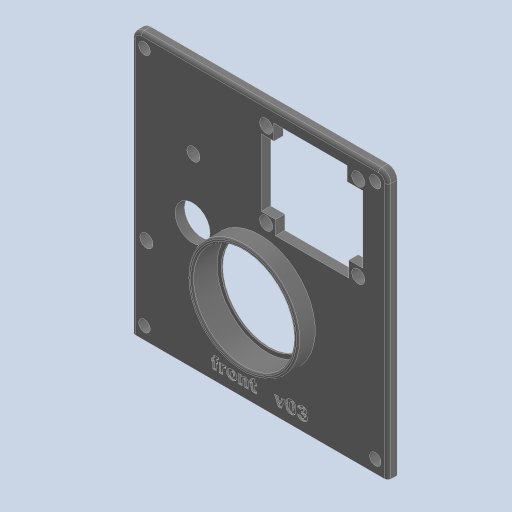
# Autodesk Inventor part: door_front_03b
Saved by Autodesk Inventor 2024.4 (Build 284460030, 460C)
## iProperties
Created: 2026-07-13
Part Number: door_front_03b
Material: Generic
Document SubType Name: Modeling
Designer: tooles01
Density: 1 g/cm^3
Appearance: Gray
d0: 3.000 mm
d1: 0.00 deg
d3: 32.500 mm
d4: 35.500 mm
d6: 0.00 deg
d11: 29.750 mm
d13: 0.00 deg
d14: 3.700 mm
d0_1: 36.000 mm
d3_1: 4.900 mm
d4_1: 3.000 mm
d5_1: 10.000 mm
d6_1: 2.000 mm
d7: 2.000 mm
d21: 30.000 mm
d22: 82.000 mm
d23: 4.000 mm
d24: 4.000 mm
d25: 4.000 mm
d26: 4.200 mm
d27: 35.000 mm
d28: 3.000 mm
d29: 4.900 mm
d32: 6.500 mm
d33: 2.000 mm
d34: 2.000 mm
d35: 10.000 mm
d37: 36.000 mm
d38: 2.000 mm
d39: 4.900 mm
d41: 4.200 mm
d48: 1.000 ul
d52: 0.00 deg
d53: 3.000 mm
d54: 34.500 mm
d55: 32.000 mm
d56: 3.000 mm
d57: 2.500 mm
d58: 27.000 mm
d59: 19.000 mm
d60: 7.000 mm
d61: 4.200 mm
d68: 55.000 mm
d69: 3.000 mm
d70: 1.000 mm
d71: 0.500 mm
d72: 40.000 mm
d73: 0.500 mm
d75: 5.000 mm
door_diameter: 36.000 mm
axle_width: 4.900 mm
axle_height: 3.100 mm
handle_height: 10.000 mm
spacing_height: 2.000 mm
spacing_width: 2.000 mm
door_diameter_1: 36.000 mm
handle_height_1: 10.000 mm
spacing_width_1: 2.000 mm
door_spacing_width_1: 2.000 mm
door_handle_height_1: 10.000 mm
door_door_diameter_1: 36.000 mm
door_axle_width_1: 4.900 mm
door_spacing_height_1: 2.000 mm
door_axle_width_2: 4.900 mm
door_axle_height_1: 3.100 mm
door_spacing_height_2: 2.000 mm
d76: 4.000 mm
d77: 9.200 mm
d78: 1.000 mm
d81: 1.000 mm
d85: 29.500 mm
d88: 27.000 mm
M3_heatset: 4.200 mm
tube_cover_length: 8.500 mm
tube_stopper_thickness: 0.500 mm
Author: tooles01
Autodesk Inventor part; units mm, degrees
ref_plane "YZ Plane" through (0, 0, 0) normal (1, 0, 0) x (0, 1, 0)
ref_plane "XZ Plane" through (0, 0, 0) normal (0, 1, 0) x (-1, 0, 0)
ref_plane "XY Plane" through (0, 0, 0) normal (0, 0, 1) x (1, 0, 0)
derived "door_03.ipt"
sketch "Sketch1: base" plane through (0, 0, 0) normal (0, 0, 1) x (1, 0, 0)
  line L0 (-41, 85) -> (41, 85)
  line L1 (41, 85) -> (41, 0)
  line L2 (41, 0) -> (-41, 0)
  line L3 (-41, 0) -> (-41, 85)
  circle A0 centre (0, 30) radius 16.25
  line L4 (-37, 81) -> (37, 81) construction
  line L5 (37, 81) -> (37, 4) construction
  line L6 (37, 4) -> (-37, 4) construction
  line L7 (-37, 4) -> (-37, 81) construction
  point P0 (0, 0)
  point P1 (0, 0)
  point P2 (0, 4)
  dimension "d3" = 32.5
  dimension "d21" = 30
  dimension "d22" = 82
  dimension "d23" = 4
  dimension "d24" = 4
  dimension "d25" = 4
  dimension "d68" = 55
  constraints: 16 end point, 6 perpendicular, 5 coincident, 2 horizontal, 2 midpoint, 2 vertical alignment, 1 centre point
  measures "d3" diameter of A0
  measures "d21" distance from line of L2 A0.centre
  measures "d22" distance of L1.end L2.end
  measures "d23" distance between parallel lines of L2 L6
  measures "d24" distance between parallel lines of L3 L7
  measures "d25" distance between parallel lines of L0 L4
  measures "d68" distance from line of L0 A0.centre
sketch "Sketch2: tube cover/stopper" plane through (0, 0, 0) normal (0, 0, 1) x (1, 0, 0)
  circle A0 centre (0, 30) radius 17.75
  circle A1 centre (0, 30) radius 14.875
  circle A2 centre (0, 30) radius 16.25 projected
  point P0 (0, 0)
  dimension "d4" = 35.5
  dimension "d11" = 29.75
  constraints: 3 coincident, 2 centre point
  measures "d4" diameter of A0
  measures "d11" diameter of A1
sketch "Sketch3: motor & door footprint" plane through (0, 0, 0) normal (0, 0, 1) x (1, 0, 0)
  circle A0 centre (-21.3026, 59.5414) radius 2.1 construction
  circle A1 centre (-36.3632, 27.9475) radius 2.1 construction
  line L0 (-21.3026, 59.5414) -> (-36.3632, 27.9475) construction
  line L1 (-19.1129, 41.8251) -> (-21.2213, 37.402)
  line L2 (-21.2213, 37.402) -> (-24.0197, 38.7359)
  line L3 (-24.0197, 38.7359) -> (-21.9112, 43.1591)
  line L4 (-21.9112, 43.1591) -> (-19.1129, 41.8251)
  line L5 (-22.9654, 40.9475) -> (-28.8329, 43.7445) construction
  line L6 (-22.8559, 45.825) -> (-26.6856, 37.7911)
  line L7 (-26.6856, 37.7911) -> (-17.6588, 33.4881)
  line L8 (-13.8291, 41.522) -> (-22.8559, 45.825)
  circle A2 centre (0, 30) radius 18
  line L9 (0, 30) -> (-24.7708, 41.8081) construction
  circle A3 centre (0, 30) radius 16.25 construction
  circle A4 centre (-20.1173, 64.1278) radius 18 construction
  line L10 (-25.6169, 46.9885) -> (-26.2234, 37.0069) construction
  line L11 (-26.2234, 37.0069) -> (-17.3397, 36.4672) construction
  line L12 (-17.3397, 36.4672) -> (-16.7333, 46.4488) construction
  line L13 (-19.0268, 41.6791) -> (-23.9177, 41.9762) construction
  line L14 (-23.9177, 41.9762) -> (-24.1058, 38.8819) construction
  line L15 (-24.1058, 38.8819) -> (-19.2148, 38.5848) construction
  line L16 (-19.2148, 38.5848) -> (-19.0268, 41.6791) construction
  line L17 (-20.1173, 64.1278) -> (-21.7816, 36.737) construction
  circle A5 centre (-21.5663, 40.2805) radius 2.45 construction
  point P0 (0, 0)
  point P1 (-20.1671, 39.6135)
  point P2 (-21.6603, 38.7334)
  point P3 (-22.6205, 38.0689)
  point P4 (-19.1208, 40.1319)
  dimension "d26" = 4.2
  dimension "d27" = 34.9999
  dimension "door_axle_height_1" = 3.1
  dimension "door_axle_width_1" = 4.9
  dimension "d32" = 6.5
  dimension "door_spacing_height_1" = 2
  dimension "door_spacing_width_1" = 2
  dimension "door_handle_height_1" = 10
  dimension "door_door_diameter_1" = 36
  dimension "door_spacing_height_2" = 2
  dimension "door_axle_width_2" = 4.9
  constraints: 36 end point, 8 midpoint, 8 perpendicular, 7 parallel, 6 point on circle, 5 centre point, 5 coincident, 4 equal length, 4 point on line, 2 equal radius, 1 collinear, 1 other
  measures "d26" diameter of A0
  measures "d27" distance of L0.start L0.end
  measures "door_axle_height_1" distance of L3.end L1.start
  measures "door_axle_width_1" distance of L1.start L1.end
  measures "d32" distance from line of A0.centre L3
  measures "door_spacing_height_1" distance between parallel lines of L6 L3
  measures "door_spacing_width_1" distance between parallel lines of L8 L4
  measures "door_handle_height_1" distance of L8.start L6.start
  measures "door_door_diameter_1" diameter of A2
  measures "door_spacing_height_2" distance between parallel lines of L11 L15
  measures "door_axle_width_2" diameter of A5
sketch "Sketch4: holes for motor mount" plane through (0, 0, 0) normal (0, 0, 1) x (1, 0, 0)
  circle A0 centre (-21.5663, 40.2805) radius 2.45 construction
  circle A1 centre (-21.5663, 40.2805) radius 5.6
  circle A2 centre (-21.5663, 40.2805) radius 4.6 construction
  point P0 (0, 0)
  point P1 (-21.3026, 59.5414)
  point P2 (-36.3632, 27.9475)
  dimension "d77" = 9.2
  dimension "d78" = 1
  constraints: 2 centre point, 2 coincident
  measures "d77" diameter of A2
  measures "d78" radial gap between concentric circles of A1 A2
sketch "Sketch6: text" plane through (0, 0, 0) normal (0, 0, 1) x (1, 0, 0)
  line L0 (-20, 7) -> (20, 7) construction
  line L1 (20, 7) -> (20, 3) construction
  line L2 (20, 3) -> (-20, 3) construction
  line L3 (-20, 3) -> (-20, 7) construction
  line L4 (-13.9634, 5.8989) -> (-13.4321, 5.8989)
  line L5 (-13.4321, 5.8989) -> (-13.4321, 5.0866)
  line L6 (-13.4321, 5.0866) -> (-13.9634, 5.0866)
  line L7 (-13.9634, 5.0866) -> (-13.9634, 3)
  line L8 (-13.9634, 3) -> (-15.076, 3)
  line L9 (-15.076, 3) -> (-15.076, 5.0866)
  line L10 (-15.076, 5.0866) -> (-15.4918, 5.0866)
  line L11 (-15.4918, 5.0866) -> (-15.4918, 5.8989)
  line L12 (-15.4918, 5.8989) -> (-15.076, 5.8989)
  line L13 (-15.076, 5.8989) -> (-15.076, 6.0298)
  spline S0 degree 2 poles (-15.076, 6.0298) (-15.076, 6.2069) (-14.999, 6.6343) (-14.7911, 6.9038) (-14.41, 7.0693) (-14.0443, 7.0693) knots 0 0 0 1 2 3 4 4 4
  spline S1 degree 2 poles (-14.0443, 7.0693) (-13.7517, 7.0693) (-13.1973, 7) knots 0 0 0 1 1 1
  line L14 (-13.1973, 7) -> (-13.3205, 6.3301)
  spline S2 degree 2 poles (-13.3205, 6.3301) (-13.5168, 6.3609) (-13.64, 6.3609) knots 0 0 0 1 1 1
  spline S3 degree 2 poles (-13.64, 6.3609) (-13.7902, 6.3609) (-13.9211, 6.2608) (-13.948, 6.153) knots 0 0 0 1 2 2 2
  spline S4 degree 2 poles (-13.948, 6.153) (-13.9634, 6.0914) (-13.9634, 5.8989) knots 0 0 0 1 1 1
  line L15 (-13.0125, 5.8989) -> (-11.9731, 5.8989)
  line L16 (-11.9731, 5.8989) -> (-11.9731, 5.4254)
  spline S5 degree 2 poles (-11.9731, 5.4254) (-11.8229, 5.7334) (-11.5034, 5.9644) (-11.2685, 5.9644) knots 0 0 0 1 2 2 2
  spline S6 degree 2 poles (-11.2685, 5.9644) (-11.0221, 5.9644) (-10.7295, 5.8104) knots 0 0 0 1 1 1
  line L17 (-10.7295, 5.8104) -> (-11.0722, 5.0212)
  spline S7 degree 2 poles (-11.0722, 5.0212) (-11.2685, 5.102) (-11.384, 5.102) knots 0 0 0 1 1 1
  spline S8 degree 2 poles (-11.384, 5.102) (-11.6035, 5.102) (-11.7228, 4.9211) knots 0 0 0 1 1 1
  spline S9 degree 2 poles (-11.7228, 4.9211) (-11.8961, 4.667) (-11.8961, 3.9702) knots 0 0 0 1 1 1
  line L18 (-11.8961, 3.9702) -> (-11.8961, 3)
  line L19 (-11.8961, 3) -> (-13.0125, 3)
  line L20 (-13.0125, 3) -> (-13.0125, 5.8989)
  spline S10 degree 2 poles (-10.6756, 4.4398) (-10.6756, 5.1059) (-9.7825, 5.9644) (-9.0202, 5.9644) knots 0 0 0 1 2 2 2
  spline S11 degree 2 poles (-9.0202, 5.9644) (-8.1501, 5.9644) (-7.7074, 5.4601) knots 0 0 0 1 1 1
  spline S12 degree 2 poles (-7.7074, 5.4601) (-7.3494, 5.052) (-7.3494, 4.4591) knots 0 0 0 1 1 1
  spline S13 degree 2 poles (-7.3494, 4.4591) (-7.3494, 3.7892) (-8.2348, 2.9346) (-9.0164, 2.9346) knots 0 0 0 1 2 2 2
  spline S14 degree 2 poles (-9.0164, 2.9346) (-9.717, 2.9346) (-10.1482, 3.2887) knots 0 0 0 1 1 1
  spline S15 degree 2 poles (-10.1482, 3.2887) (-10.6756, 3.7276) (-10.6756, 4.4398) knots 0 0 0 1 1 1
  spline S16 degree 2 poles (-9.563, 4.4437) (-9.563, 4.0549) (-9.2512, 3.6853) (-9.0125, 3.6853) knots 0 0 0 1 2 2 2
  spline S17 degree 2 poles (-9.0125, 3.6853) (-8.7738, 3.6853) (-8.4658, 4.051) (-8.4658, 4.4552) knots 0 0 0 1 2 2 2
  spline S18 degree 2 poles (-8.4658, 4.4552) (-8.4658, 4.8287) (-8.7777, 5.1983) (-9.0048, 5.1983) knots 0 0 0 1 2 2 2
  spline S19 degree 2 poles (-9.0048, 5.1983) (-9.2474, 5.1983) (-9.563, 4.8248) (-9.563, 4.4437) knots 0 0 0 1 2 2 2
  line L21 (-6.8104, 5.8989) -> (-5.7748, 5.8989)
  line L22 (-5.7748, 5.8989) -> (-5.7748, 5.4254)
  spline S20 degree 2 poles (-5.7748, 5.4254) (-5.5438, 5.718) (-5.0664, 5.9644) (-4.7276, 5.9644) knots 0 0 0 1 2 2 2
  spline S21 degree 2 poles (-4.7276, 5.9644) (-4.2656, 5.9644) (-3.7459, 5.4139) (-3.7459, 4.8441) knots 0 0 0 1 2 2 2
  line L23 (-3.7459, 4.8441) -> (-3.7459, 3)
  line L24 (-3.7459, 3) -> (-4.8624, 3)
  line L25 (-4.8624, 3) -> (-4.8624, 4.5938)
  spline S22 degree 2 poles (-4.8624, 4.5938) (-4.8624, 4.8672) (-5.0626, 5.0943) (-5.2474, 5.0943) knots 0 0 0 1 2 2 2
  spline S23 degree 2 poles (-5.2474, 5.0943) (-5.4475, 5.0943) (-5.6978, 4.7902) (-5.6978, 4.3936) knots 0 0 0 1 2 2 2
  line L26 (-5.6978, 4.3936) -> (-5.6978, 3)
  line L27 (-5.6978, 3) -> (-6.8104, 3)
  line L28 (-6.8104, 3) -> (-6.8104, 5.8989)
  line L29 (-1.7401, 7) -> (-1.7401, 5.8989)
  line L30 (-1.7401, 5.8989) -> (-1.128, 5.8989)
  line L31 (-1.128, 5.8989) -> (-1.128, 5.0866)
  line L32 (-1.128, 5.0866) -> (-1.7401, 5.0866)
  line L33 (-1.7401, 5.0866) -> (-1.7401, 4.0587)
  spline S24 degree 2 poles (-1.7401, 4.0587) (-1.7401, 3.8739) (-1.7055, 3.8123) knots 0 0 0 1 1 1
  spline S25 degree 2 poles (-1.7055, 3.8123) (-1.6516, 3.7199) (-1.513, 3.7199) knots 0 0 0 1 1 1
  spline S26 degree 2 poles (-1.513, 3.7199) (-1.3898, 3.7199) (-1.1704, 3.7892) knots 0 0 0 1 1 1
  line L34 (-1.1704, 3.7892) -> (-1.0895, 3.0231)
  spline S27 degree 2 poles (-1.0895, 3.0231) (-1.5014, 2.9346) (-1.8595, 2.9346) knots 0 0 0 1 1 1
  spline S28 degree 2 poles (-1.8595, 2.9346) (-2.2714, 2.9346) (-2.6641, 3.1463) (-2.8527, 3.5813) (-2.8527, 4.0664) knots 0 0 0 1 2 3 3 3
  line L35 (-2.8527, 4.0664) -> (-2.8527, 5.0866)
  line L36 (-2.8527, 5.0866) -> (-3.2608, 5.0866)
  line L37 (-3.2608, 5.0866) -> (-3.2608, 5.8989)
  line L38 (-3.2608, 5.8989) -> (-2.8527, 5.8989)
  line L39 (-2.8527, 5.8989) -> (-2.8527, 6.4302)
  line L40 (-2.8527, 6.4302) -> (-1.7401, 7)
  line L41 (4.666, 5.8989) -> (5.821, 5.8989)
  line L42 (5.821, 5.8989) -> (6.3869, 4.0626)
  line L43 (6.3869, 4.0626) -> (6.9682, 5.8989)
  line L44 (6.9682, 5.8989) -> (8.0885, 5.8989)
  line L45 (8.0885, 5.8989) -> (6.8566, 3)
  line L46 (6.8566, 3) -> (5.871, 3)
  line L47 (5.871, 3) -> (4.666, 5.8989)
  spline S29 degree 2 poles (8.3041, 5.0173) (8.3041, 6.1569) (9.1242, 7.0693) (9.9634, 7.0693) knots 0 0 0 1 2 2 2
  spline S30 degree 2 poles (9.9634, 7.0693) (10.3677, 7.0693) (10.8835, 6.8691) (11.2108, 6.5496) (11.3994, 6.1992) (11.4572, 5.9644) knots 0 0 0 1 2 3 4 4 4
  spline S31 degree 2 poles (11.4572, 5.9644) (11.5688, 5.5178) (11.5688, 5.0289) knots 0 0 0 1 1 1
  spline S32 degree 2 poles (11.5688, 5.0289) (11.5688, 3.9394) (10.8335, 2.9307) (9.9326, 2.9307) knots 0 0 0 1 2 2 2
  spline S33 degree 2 poles (9.9326, 2.9307) (9.4283, 2.9307) (8.8085, 3.2541) (8.6083, 3.5659) knots 0 0 0 1 2 2 2
  spline S34 degree 2 poles (8.6083, 3.5659) (8.4658, 3.7854) (8.3041, 4.5515) (8.3041, 5.0173) knots 0 0 0 1 2 2 2
  spline S35 degree 2 poles (9.4052, 5.0135) (9.4052, 4.2474) (9.6747, 3.6891) (9.9288, 3.6891) knots 0 0 0 1 2 2 2
  spline S36 degree 2 poles (9.9288, 3.6891) (10.0982, 3.6891) (10.3484, 3.9278) (10.4639, 4.4398) (10.4639, 4.9827) knots 0 0 0 1 2 3 3 3
  spline S37 degree 2 poles (10.4639, 4.9827) (10.4639, 5.7796) (10.1944, 6.3301) (9.9249, 6.3301) knots 0 0 0 1 2 2 2
  spline S38 degree 2 poles (9.9249, 6.3301) (9.6516, 6.3301) (9.4052, 5.7719) (9.4052, 5.0135) knots 0 0 0 1 2 2 2
  line L48 (13.1126, 5.845) -> (12.0616, 6.0337)
  spline S39 degree 2 poles (12.0616, 6.0337) (12.1925, 6.5342) (12.9355, 7.0693) (13.6169, 7.0693) knots 0 0 0 1 2 2 2
  spline S40 degree 2 poles (13.6169, 7.0693) (14.4023, 7.0693) (15.0991, 6.4841) (15.0991, 6.0452) knots 0 0 0 1 2 2 2
  spline S41 degree 2 poles (15.0991, 6.0452) (15.0991, 5.7834) (14.8142, 5.3638) (14.5255, 5.206) knots 0 0 0 1 2 2 2
  spline S42 degree 2 poles (14.5255, 5.206) (14.7603, 5.1482) (14.8835, 5.0712) knots 0 0 0 1 1 1
  spline S43 degree 2 poles (14.8835, 5.0712) (15.0837, 4.948) (15.3032, 4.5476) (15.3032, 4.2705) knots 0 0 0 1 2 2 2
  spline S44 degree 2 poles (15.3032, 4.2705) (15.3032, 3.9201) (14.9374, 3.2772) (14.2522, 2.9307) (13.6901, 2.9307) knots 0 0 0 1 2 3 3 3
  spline S45 degree 2 poles (13.6901, 2.9307) (13.1473, 2.9307) (12.5159, 3.1886) (12.1078, 3.6814) (12, 4.0549) knots 0 0 0 1 2 3 3 3
  line L49 (12, 4.0549) -> (13.1126, 4.2012)
  spline S46 degree 2 poles (13.1126, 4.2012) (13.1781, 3.8662) (13.4514, 3.6083) (13.6631, 3.6083) knots 0 0 0 1 2 2 2
  spline S47 degree 2 poles (13.6631, 3.6083) (13.8864, 3.6083) (14.1829, 3.9355) (14.1829, 4.2089) knots 0 0 0 1 2 2 2
  spline S48 degree 2 poles (14.1829, 4.2089) (14.1829, 4.4899) (13.898, 4.794) (13.6516, 4.794) knots 0 0 0 1 2 2 2
  spline S49 degree 2 poles (13.6516, 4.794) (13.5207, 4.794) (13.2936, 4.7286) knots 0 0 0 1 1 1
  line L50 (13.2936, 4.7286) -> (13.3513, 5.5255)
  spline S50 degree 2 poles (13.3513, 5.5255) (13.4437, 5.5101) (13.4937, 5.5101) knots 0 0 0 1 1 1
  spline S51 degree 2 poles (13.4937, 5.5101) (13.7132, 5.5101) (14.0058, 5.7873) (14.0058, 5.9798) knots 0 0 0 1 2 2 2
  spline S52 degree 2 poles (14.0058, 5.9798) (14.0058, 6.1607) (13.7863, 6.3802) (13.5977, 6.3802) knots 0 0 0 1 2 2 2
  spline S53 degree 2 poles (13.5977, 6.3802) (13.4013, 6.3802) (13.155, 6.1415) (13.1126, 5.845) knots 0 0 0 1 2 2 2
  point P0 (0, 0)
  point P1 (0, 3)
  point P2 (-20, 5)
  dimension "d72" = 40
  dimension "d75" = 5
  dimension "d76" = 4
  constraints: 2 midpoint, 1 horizontal, 1 vertical alignment, 2 other
  measures "d72" distance of L0.start L0.end
  measures "d75" vertical distance of point (0, 0) point (-20, 5)
  measures "d76" distance of L2.end L0.start
extrude "Ex1: base" add sketch "Sketch1: base" along normal blind 3
extrude "Ex2: tube cover" add sketch "Sketch2: tube cover/stopper" along normal blind 8.5 contours A0
sketch "Sketch5: PCB footprint" plane through (0, 0, 0) normal (0, 0, 1) x (1, 0, 0)
  line L0 (-0.5, 81) -> (34, 81)
  line L1 (34, 81) -> (34, 49)
  line L2 (34, 49) -> (-0.5, 49)
  line L3 (-0.5, 49) -> (-0.5, 81)
  circle A0 centre (2, 79) radius 1.5
  circle A1 centre (31.5, 79) radius 1.5
  circle A2 centre (2, 52) radius 1.5
  circle A3 centre (31.5, 52) radius 1.5
  line L4 (2, 79) -> (31.5, 79) construction
  line L5 (31.5, 79) -> (31.5, 52) construction
  line L6 (31.5, 52) -> (2, 52) construction
  line L7 (2, 52) -> (2, 79) construction
  circle A4 centre (0, 30) radius 17.75 projected
  line L8 (41, 0) -> (41, 85) projected
  circle A5 centre (2, 79) radius 0.5 construction
  circle A6 centre (31.5, 79) radius 0.5 construction
  circle A7 centre (31.5, 52) radius 0.5 construction
  circle A8 centre (2, 52) radius 0.5 construction
  point P0 (0, 0)
  point P1 (16.75, 79)
  point P2 (16.75, 81)
  dimension "d53" = 3
  dimension "d54" = 34.5
  dimension "d55" = 32
  dimension "d56" = 3
  dimension "d57" = 2.5
  dimension "d58" = 27
  dimension "d59" = 19
  dimension "d60" = 7
  dimension "d81" = 1
  dimension "d85" = 29.5
  dimension "d88" = 27
  constraints: 16 end point, 8 centre point, 6 equal radius, 6 perpendicular, 5 coincident, 3 vertical alignment, 2 horizontal, 2 horizontal alignment, 2 midpoint
  measures "d53" diameter of A0
  measures "d54" distance of L0.start L0.end
  measures "d55" distance of L2.end L0.start
  measures "d56" distance from line of L2 A2.centre
  measures "d57" distance from line of A2.centre L3
  measures "d58" distance of L6.end L4.start
  measures "d59" distance from line of A4.centre L2
  measures "d60" distance between parallel lines of L8 L1
  measures "d81" diameter of A5
  measures "d85" distance of A5.centre A6.centre
  measures "d88" distance of A6.centre A7.centre
extrude "Ex3: tube stopper" add sketch "Sketch2: tube cover/stopper" along normal blind 0.5 contours A2
hole "Hole1: mounting (M3 thru holes)" at (-37, 81, 0) at (37, 81, 0) at (-37, 4, 0) at (37, 4, 0) direction (0, 0, 1) diameter 3.7 end through all
hole "Hole2: motor mount (M3 heat-set)" at (-21.3026, 59.5414, 0) at (-36.3632, 27.9475, 0) direction (0, 0, 1) diameter 4.2 end through all
extrude "Ex4: hole for motor" cut sketch "Sketch4: holes for motor mount" along normal through all both and the other way through all
hole "Hole3: PCB holes (M3 heat-set)" at (31.5, 79, 0) at (2, 79, 0) at (2, 52, 0) at (31.5, 52, 0) direction (0, 0, 1) diameter 4.2 end through all
sketch "Sketch: space for PCB footprint" plane through (0, 0, 0) normal (0, 0, 1) x (1, 0, 0)
  line L0 (28, 78.5) -> (28, 78.5)
  line L1 (28, 78.5) -> (28, 76.5)
  line L2 (28.5, 50) -> (5, 50)
  line L3 (4.5, 81) -> (28, 81)
  line L4 (28, 81) -> (28, 78.5)
  line L5 (28, 76.5) -> (33, 76.5)
  line L6 (33, 76.5) -> (33, 55)
  line L7 (33, 55) -> (28.5, 55)
  line L8 (-0.5, 81) -> (34, 81) construction
  line L9 (-0.5, 49) -> (-0.5, 81) construction
  line L10 (34, 81) -> (34, 49) construction
  line L11 (34, 49) -> (-0.5, 49) construction
  circle A0 centre (31.5, 52) radius 1.5 construction
  circle A1 centre (2, 52) radius 1.5 construction
  circle A2 centre (2, 79) radius 1.5 construction
  circle A3 centre (31.5, 79) radius 1.5 construction
  line L12 (4.5, 76) -> (0.5, 76)
  line L13 (0.5, 76) -> (0.5, 54.5)
  line L14 (0.5, 54.5) -> (5, 54.5)
  line L15 (28.5, 55) -> (28.5, 50)
  line L16 (5, 54.5) -> (5, 50)
  line L17 (4.5, 76) -> (4.5, 79.5)
  line L18 (4.5, 81) -> (4.5, 79.5)
  line L19 (4.5, 79.5) -> (4.5, 79.5)
  point P0 (0, 0)
  point P1 (28, 78.5)
  dimension "d105" = 23.5
  dimension "d106" = 2.5
  dimension "d113" = 3
  dimension "d114" = 3
  dimension "d115" = 2.5
  dimension "d116" = 1
  dimension "d117" = 1
  dimension "d120" = 3.5
  dimension "d121" = 1
  dimension "d122" = 3
  dimension "d123" = 3.5
  dimension "d125" = 3
  dimension "d126" = 2.5
  dimension "d128" = 2.5
  dimension "d131" = 0.5
  dimension "d132" = 2
  dimension "d133" = 0.5
  dimension "d134" = 2.5
  constraints: 33 end point, 13 perpendicular, 1 horizontal
  measures "d105" distance of L3.start L3.end
  measures "d106" distance from line of A3.centre L5
  measures "d113" distance from line of A0.centre L7
  measures "d114" distance from line of L12 A2.centre
  measures "d115" distance from line of L14 A1.centre
  measures "d116" distance between parallel lines of L10 L6
  measures "d117" distance between parallel lines of L9 L13
  measures "d120" distance from line of L4 A3.centre
  measures "d121" distance between parallel lines of L11 L2
  measures "d122" distance from line of L15 A0.centre
  measures "d123" distance from line of A3.centre L1
  measures "d125" distance from line of A1.centre L16
  measures "d126" distance from line of A2.centre L17
  measures "d128" distance of L3.end L0.start
  measures "d131" distance from line of A3.centre L0
  measures "d132" distance from line of A2.centre L3
  measures "d133" distance from line of A2.centre L19
  measures "d134" distance from line of A2.centre L18
extrude "Ex: space for PCB back" cut sketch "Sketch: space for PCB footprint" along normal through all both and the other way through all
extrude "Ex5: text" cut sketch "Sketch6: text" against normal blind 0.5 from surface at 3
fillet "Fillet1" radius 3 2 edges at (41, 85, 1.5) (-41, 85, 1.5)
fillet "Fillet2" radius 1 5 edges at (40.1213, 84.1213, 3) (0, 85, 3) (-40.1213, 84.1213, 3) (-41, 41, 3) (41, 41, 3)
fillet "Fillet3" radius 0.5 2 edges at (-16.25, 30, 8.5) (-17.75, 30, 8.5)
equation "\"d24\" = d23"
equation "\"d25\" = d23"
equation "\"M3_heatset\" = 4.2"
equation "\"length_of_tube_pressfit\" = 8"
body "Solid1"
